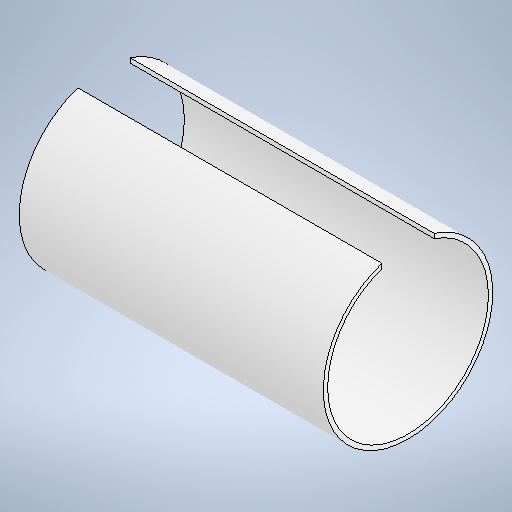
# Autodesk Inventor part: joint4_bush
Saved by Autodesk Inventor 2025.3 (Build 293356030, 356C)
## iProperties
Created: 2025-11-11
Part Number: joint4_bush
Material: PLA filament
Document SubType Name: Modeling
Designer: MSI
Mass: 1.1253 g
Surface Area: 38.4146 cm^2
Volume: 0.93775 cm^3
Density: 1.2 g/cm^3
Appearance: 일반
Author: MSI
Autodesk Inventor part; units mm, degrees
ref_plane "YZ Plane" through (0, 0, 0) normal (1, 0, 0) x (0, 1, 0)
ref_plane "XZ Plane" through (0, 0, 0) normal (0, 1, 0) x (-1, 0, 0)
ref_plane "XY Plane" through (0, 0, 0) normal (0, 0, 1) x (1, 0, 0)
sketch "스케치1" plane through (0, 0, 0) normal (1, 0, 0) x (0, 1, 0)
  circle A0 centre (0, 0) radius 9.75
  circle A1 centre (0, 0) radius 9.25
  line L0 (12.25, 3) -> (7.25, 3)
  line L1 (7.25, 3) -> (7.25, -3)
  line L2 (7.25, -3) -> (12.25, -3)
  line L3 (12.25, -3) -> (12.25, 3)
  line L4 (12.25, 3) -> (7.25, -3) construction
  line L5 (7.25, 3) -> (12.25, -3) construction
  point P0 (9.75, 0)
  point P1 (7.25, 0)
  point P2 (9.277, -3)
  point P3 (8.75, -3)
  point P4 (8.75, 3)
  point P5 (9.277, 3)
  dimension "d0" = 19.5
  dimension "d1" = 18.5
  dimension "d2" = 6
  dimension "d3" = 5
  constraints: 12 end point, 3 midpoint, 2 coincident, 2 parallel, 1 centre point, 1 horizontal, 1 horizontal alignment, 1 perpendicular, 3 other
  measures "d1" diameter of A1
  measures "d2" distance of L2.end L0.start
  measures "d3" distance of L1.end L2.end
extrude "돌출1" add sketch "스케치1" along normal blind 35 contours L0 A1 L2 A0 picked at (-9.5112, -0.3759)
